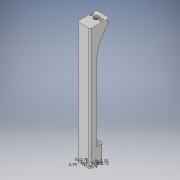
# Autodesk Inventor part: Camera Mount 30mm
Saved by Autodesk Inventor 2019 (Build 230136000, 136)
## iProperties
Created: 2020-02-21
Part Number: Camera Mount 30mm
Material: Generic
Document SubType Name: Modeling
Designer: close
Density: 1 g/cm^3
Appearance: Default
Author: close
Autodesk Inventor part; units mm, degrees
ref_plane "YZ Plane" through (0, 0, 0) normal (1, 0, 0) x (0, 1, 0)
ref_plane "XZ Plane" through (0, 0, 0) normal (0, 1, 0) x (-1, 0, 0)
sketch "Sketch1" plane through (0, 0, 0) normal (0, 1, 0) x (-1, 0, 0)
  line L0 (6, 8) -> (-6, 8)
  line L1 (-8, 6) -> (-8, -6)
  line L2 (-6, -8) -> (6, -8)
  line L3 (8, -6) -> (8, 6)
  arc A0 (8, 6) -> (6, 8) centre (6, 6) ccw
  arc A1 (-6, 8) -> (-8, 6) centre (-6, 6) ccw
  arc A2 (-8, -6) -> (-6, -8) centre (-6, -6) ccw
  arc A3 (6, -8) -> (8, -6) centre (6, -6) ccw
  point P0 (0, 0)
  point P1 (8, 8)
  point P2 (-8, 8)
  point P3 (8, -8)
  dimension "d0" = 16
  dimension "d1" = 16
  dimension "d2" = 8
  dimension "d3" = 8
  dimension "d4" = 2
  constraints: 8 end point, 8 point on circle, 8 tangent, 6 point on line, 4 centre point, 3 equal radius, 2 parallel, 1 horizontal, 1 perpendicular
  measures "d0" distance of point (8, -8) point (8, 8)
  measures "d1" distance of point (8, 8) point (-8, 8)
  measures "d2" distance from line of L0 point (0, 0)
  measures "d3" distance from line of point (0, 0) L3
  measures "d4" radius of A0
extrude "Extrusion1" add sketch "Sketch1" along normal blind 150
sketch "Sketch2" plane through (0, 0, 0) normal (0, -1, 0) x (1, 0, 0)
  line L0 (-6, 5.875) -> (-6, 3.125) construction
  line L1 (-7.375, 5.875) -> (-7.375, 3.125)
  line L2 (-4.625, 3.125) -> (-4.625, 5.875)
  arc A0 (-4.625, 5.875) -> (-7.375, 5.875) centre (-6, 5.875) ccw
  arc A1 (-7.375, 3.125) -> (-4.625, 3.125) centre (-6, 3.125) ccw
  line L3 (6, -3.125) -> (6, -5.875) construction
  line L4 (4.625, -3.125) -> (4.625, -5.875)
  line L5 (7.375, -5.875) -> (7.375, -3.125)
  arc A2 (7.375, -3.125) -> (4.625, -3.125) centre (6, -3.125) ccw
  arc A3 (4.625, -5.875) -> (7.375, -5.875) centre (6, -5.875) ccw
  point P0 (0, 0)
  point P1 (0, 0)
  point P2 (-6, 4.5)
  point P3 (6, -4.5)
  dimension "d7" = 2.75
  dimension "d8" = 12
  dimension "d9" = 6
  dimension "d10" = 9
  dimension "d11" = 4.5
  dimension "d12" = 2.75
  dimension "d13" = 2.75
  dimension "d14" = 2.75
  constraints: 16 end point, 8 point on circle, 8 tangent, 4 centre point, 3 parallel, 2 midpoint, 1 coincident, 1 vertical
  measures "d7" distance between parallel lines of L2 L1
  measures "d8" distance from line of point (6, -4.5) L0
  measures "d9" distance from line of point (0, 0) L0
  measures "d10" vertical distance of point (6, -4.5) point (-6, 4.5)
  measures "d11" vertical distance of point (0, 0) point (6, -4.5)
  measures "d12" distance of L0.start L0.end
  measures "d13" distance of L3.start L3.end
  measures "d14" distance between parallel lines of L5 L4
extrude "Extrusion2" cut sketch "Sketch2" against normal blind 2.5
sketch "Sketch3" plane through (0, 150, 0) normal (0, 1, 0) x (1, 0, 0)
  line L0 (-6, 9.5) -> (-6, 6.5) construction
  line L1 (-6.6, 9.5) -> (-6.6, 6.5)
  line L2 (-5.4, 6.5) -> (-5.4, 9.5)
  arc A0 (-5.4, 9.5) -> (-6.6, 9.5) centre (-6, 9.5) ccw
  arc A1 (-6.6, 6.5) -> (-5.4, 6.5) centre (-6, 6.5) ccw
  line L3 (6, 9.5) -> (6, 6.5) construction
  line L4 (5.4, 9.5) -> (5.4, 6.5)
  line L5 (6.6, 6.5) -> (6.6, 9.5)
  arc A2 (6.6, 9.5) -> (5.4, 9.5) centre (6, 9.5) ccw
  arc A3 (5.4, 6.5) -> (6.6, 6.5) centre (6, 6.5) ccw
  line L6 (-6, 8) -> (6, 8) construction
  line L7 (6, 8) -> (-6, 8) projected
  circle A4 centre (0, 0) radius 3.378 construction
  circle A5 centre (0, 8) radius 3.494
  dimension "d25" = 0.6
  dimension "d26" = 0.6
  dimension "d27" = 3
  dimension "d30" = 12
  dimension "d32" = 3
  dimension "d35" = 6
  dimension "d36" = 0
  constraints: 18 end point, 8 point on circle, 8 tangent, 5 centre point, 4 equal length, 3 midpoint, 1 vertical
  measures "d25" radius of A0
  measures "d26" radius of A2
  measures "d27" distance of L3.start L3.end
  measures "d30" distance between parallel lines of L3 L0
  measures "d32" distance of L0.start L0.end
  measures "d35" distance from line of A4.centre L0
  measures "d36" distance between parallel lines of L6 L7
extrude "Extrusion3" add sketch "Sketch3" along normal blind 1.5 contours A0 L2 A1 L1 | L4 A2 L5 A3
ref_plane "Work Plane1" through (6, 0, -16) normal (0, 0, -1) x (-1, 0, 0)
sketch "Sketch4" plane through (6, 0, -16) normal (0, 0, -1) x (-1, 0, 0)
  line L0 (-2, 0) -> (-2, 150) projected
  line L1 (14, 0) -> (14, 150) projected
  line L2 (-2, 150) -> (14, 150)
  line L3 (14, 150) -> (14, 135)
  line L4 (14, 135) -> (-2, 135)
  line L5 (-2, 135) -> (-2, 150)
  point P0 (6, 0)
  dimension "d38" = 15
  constraints: 8 end point, 2 parallel, 1 horizontal, 1 perpendicular, 1 point on line
  measures "d38" distance between parallel lines of L4 L2
extrude "Extrusion4" add sketch "Sketch4" against normal blind 10
fillet "Fillet1" radius 2 2 edges at (8, 142.5, -16) (-8, 142.5, -16)
sketch "Sketch5" plane through (8, 0, 6) normal (1, 0, 0) x (0, 0, -1)
  line L0 (22, 135) -> (22, 150) projected
  line L1 (22, 146) -> (6, 146)
  line L2 (6, 146) -> (6, 20)
  line L3 (6, 20) -> (22, 20)
  line L4 (22, 20) -> (22, 146)
  line L5 (-2, 0) -> (-2, 150) projected
  line L6 (0, 150) -> (20, 150) projected
  point P0 (6, 0)
  dimension "d42" = 8
  dimension "d43" = 20
  dimension "d44" = 4
  constraints: 8 end point, 2 parallel, 1 horizontal, 1 perpendicular, 1 point on line
  measures "d42" distance between parallel lines of L5 L2
  measures "d43" distance from line of L5.start L3
  measures "d44" distance between parallel lines of L1 L6
extrude "Extrusion5" cut sketch "Sketch5" against normal up to surface (16 mm away)
hole "Hole2" at (0, 150, -8) direction (0, -1, 0) diameter 6.756 depth 7 clearance for "Flat Head Machine Screw (82)" size "1/4" standard "Ansi Unified Screw Threads"
sketch "Sketch6" plane through (8, 0, 6) normal (1, 0, 0) x (0, 0, -1)
  line L0 (22, 146) -> (20, 146) projected
  arc A0 (22, 146) -> (6, 109.9866) centre (54.5302, 109.9866) ccw
  line L1 (20, 146) -> (6, 146) projected
  line L2 (6, 109.9866) -> (6, 146)
  line L3 (6, 146) -> (22, 146)
  point P0 (6, 0)
  constraints: 4 end point, 2 point on circle, 1 centre point, 1 collinear, 1 vertical
extrude "Extrusion6" add sketch "Sketch6" against normal up to surface (16 mm away)
sketch "Sketch7" plane through (0, 150, 0) normal (0, 1, 0) x (1, 0, 0)
  circle A0 centre (0, 8) radius 3.378 construction
  arc A1 (-6, 16) -> (-8, 14) centre (-6, 14) ccw projected
  line L0 (-8, 14) -> (-8, -6) projected
  arc A2 (-8, -6) -> (-6, -8) centre (-6, -6) ccw projected
  line L1 (-6, -8) -> (6, -8) projected
  arc A3 (6, -8) -> (8, -6) centre (6, -6) ccw projected
  line L2 (8, -6) -> (8, 14) projected
  arc A4 (8, 14) -> (6, 16) centre (6, 14) ccw projected
  line L3 (6, 16) -> (-6, 16) projected
  line L4 (6.6, 6.5) -> (6.6, 9.5) construction
  arc A5 (5.4, 6.5) -> (6.6, 6.5) centre (6, 6.5) ccw construction
  line L5 (5.4, 9.5) -> (5.4, 6.5) construction
  arc A6 (6.6, 9.5) -> (5.4, 9.5) centre (6, 9.5) ccw construction
  line L6 (-6.6, 9.5) -> (-6.6, 6.5) construction
  arc A7 (-5.4, 9.5) -> (-6.6, 9.5) centre (-6, 9.5) ccw construction
  line L7 (-5.4, 9.5) -> (-5.4, 6.5) construction
  arc A8 (-6.6, 6.5) -> (-5.4, 6.5) centre (-6, 6.5) ccw construction
  line L8 (-17.4625, -22.225) -> (15.875, -22.225)
  line L9 (15.875, -22.225) -> (15.875, 22.225)
  line L10 (15.875, 22.225) -> (-17.4625, 22.225)
  line L11 (-17.4625, 22.225) -> (-17.4625, -22.225)
  point P0 (0, 0)
  constraints: 8 end point, 2 parallel, 1 horizontal, 1 perpendicular
extrude "Extrusion7" cut sketch "Sketch7" against normal blind 10
sketch "Sketch8" plane through (6, 0, -16) normal (0, 0, -1) x (-1, 0, 0)
  line L0 (0, 146) -> (12, 146) projected
  line L1 (14, 109.9866) -> (-2, 109.9866) projected
  line L2 (0, 146) -> (12, 146)
  line L3 (12, 146) -> (12, 109.9866)
  line L4 (12, 109.9866) -> (0, 109.9866)
  line L5 (0, 109.9866) -> (0, 146)
  line L6 (-2, 109.9866) -> (-2, 144.0871) projected
  line L7 (14, 109.9866) -> (14, 144.0871) projected
  point P0 (6, 0)
  dimension "d68" = 2
  dimension "d69" = 2
  constraints: 8 end point, 2 parallel, 2 point on line, 1 horizontal, 1 perpendicular
  measures "d68" distance between parallel lines of L6 L5
  measures "d69" distance between parallel lines of L7 L3
extrude "Extrusion8" cut sketch "Sketch8" against normal up to surface (16 mm away)
hole "Hole3" at (0, 0, 0) direction (0, 1, 0) diameter 5.4 depth 40
equation "\"d1\" = d0"
equation "\"d2\" = 0.5 * d0"
equation "\"d3\" = d2"
equation "\"d9\" = 0.5 * d8"
equation "\"d11\" = 0.5 * d10"
equation "\"d12\" = d7"
equation "\"d13\" = d7"
equation "\"d14\" = d7"
equation "\"d26\" = d25"
equation "\"d27\" = d32"
equation "\"d35\" = 0.5 * d30"
equation "\"d69\" = d68"
body "Solid1"
